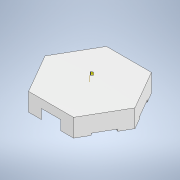
# Autodesk Inventor part: Hexagone
Saved by Autodesk Inventor 2020 (Build 240168000, 168)
## iProperties
Created: 2020-04-08
Part Number: Hexagone
Material: PVC-Piping
Document SubType Name: Modeling
Designer: Samuele
Density: 1.4 g/cm^3
Appearance: Smooth - White
Author: Samuele
## iProperties of the stored document _3DPrint.ipt
Created: 2020-04-24
Part Number: _3DPrint
Material: Generic
Document SubType Name: Modeling
Designer: Samuele
Density: 1 g/cm^3
Appearance: Default
Author: Samuele
Autodesk Inventor part; units mm, degrees
ref_plane "YZ Plane" through (0, 0, 0) normal (1, 0, 0) x (0, 1, 0)
ref_plane "XZ Plane" through (0, 0, 0) normal (0, 1, 0) x (-1, 0, 0)
ref_plane "XY Plane" through (0, 0, 0) normal (0, 0, 1) x (1, 0, 0)
sketch "Sketch6" plane through (0, 0, 0) normal (0, 1, 0) x (-1, 0, 0)
  circle A0 centre (32.5, -48.5) radius 70
  line L0 (102.5, -48.5) -> (67.5, -109.1218)
  line L1 (67.5, -109.1218) -> (-2.5, -109.1218)
  line L2 (-2.5, -109.1218) -> (-37.5, -48.5)
  line L3 (-37.5, -48.5) -> (-2.5, 12.1218)
  line L4 (-2.5, 12.1218) -> (67.5, 12.1218)
  line L5 (67.5, 12.1218) -> (102.5, -48.5)
  line L6 (32.5, 12.1218) -> (47.5, 12.1218)
  line L7 (47.5, 12.1218) -> (47.5, 5.6218)
  line L8 (47.5, 5.6218) -> (17.5, 5.6218)
  line L9 (17.5, 5.6218) -> (17.5, 12.1218)
  line L10 (47.5, 5.6218) -> (56.6924, 5.6218) construction
  line L11 (17.5, 8.8718) -> (20, 8.8718)
  line L12 (47.5, 8.8718) -> (45, 8.8718)
  line L13 (45, 8.8718) -> (45, 10.1218)
  line L14 (45, 10.1218) -> (20, 10.1218)
  line L15 (20, 10.1218) -> (20, 7.6218)
  line L16 (20, 7.6218) -> (45, 7.6218)
  line L17 (45, 7.6218) -> (45, 10.1218)
  line L18 (47.5, 5.6218) -> (56.6924, 5.6218)
  line L19 (17.5, 5.6218) -> (11, 5.6218)
  line L20 (17.5, 12.1218) -> (11, 5.6218)
  line L21 (17.5, 12.1218) -> (26.6924, 12.1218) construction
  line L22 (47.5, 12.1218) -> (54, 5.6218)
  line L23 (85, -18.1891) -> (77.5, -5.1987)
  line L24 (77.5, -5.1987) -> (71.8708, -8.4487)
  line L25 (71.8708, -8.4487) -> (86.8708, -34.4295)
  line L26 (86.8708, -34.4295) -> (92.5, -31.1795)
  line L27 (71.8708, -8.4487) -> (67.2746, -0.4879) construction
  line L28 (89.6854, -32.8045) -> (88.4354, -30.6394)
  line L29 (74.6854, -6.8237) -> (75.9354, -8.9888)
  line L30 (75.9354, -8.9888) -> (77.0179, -8.3638)
  line L31 (77.0179, -8.3638) -> (89.5179, -30.0144)
  line L32 (89.5179, -30.0144) -> (87.3529, -31.2644)
  line L33 (87.3529, -31.2644) -> (74.8529, -9.6138)
  line L34 (74.8529, -9.6138) -> (77.0179, -8.3638)
  line L35 (71.8708, -8.4487) -> (67.2746, -0.4879)
  line L36 (86.8708, -34.4295) -> (90.1208, -40.0587)
  line L37 (92.5, -31.1795) -> (90.1208, -40.0587)
  line L38 (92.5, -31.1795) -> (87.9038, -23.2187) construction
  line L39 (77.5, -5.1987) -> (68.6208, -2.8196)
  line L40 (71.8708, -88.5513) -> (67.2746, -96.5121) construction
  line L41 (74.6854, -90.1763) -> (75.9354, -88.0112)
  line L42 (74.8529, -87.3862) -> (77.0179, -88.6362)
  line L43 (77.5, -91.8013) -> (71.8708, -88.5513)
  line L44 (77.5, -91.8013) -> (68.6208, -94.1804)
  line L45 (71.8708, -88.5513) -> (67.2746, -96.5121)
  line L46 (77.0179, -88.6362) -> (89.5179, -66.9856)
  line L47 (87.3529, -65.7356) -> (74.8529, -87.3862)
  line L48 (71.8708, -88.5513) -> (86.8708, -62.5705)
  line L49 (89.5179, -66.9856) -> (87.3529, -65.7356)
  line L50 (89.6854, -64.1955) -> (88.4354, -66.3606)
  line L51 (86.8708, -62.5705) -> (92.5, -65.8205)
  line L52 (86.8708, -62.5705) -> (90.1208, -56.9413)
  line L53 (92.5, -65.8205) -> (90.1208, -56.9413)
  line L54 (94.9944, -48.5) -> (63.7472, -102.6218)
  line L55 (63.7472, -102.6218) -> (1.2528, -102.6218)
  line L56 (1.2528, -102.6218) -> (-29.9944, -48.5)
  line L57 (-29.9944, -48.5) -> (1.2528, 5.6218)
  line L58 (1.2528, 5.6218) -> (63.7472, 5.6218)
  line L59 (63.7472, 5.6218) -> (94.9944, -48.5)
  line L60 (74.8529, -87.3862) -> (73.1208, -86.3862)
  line L61 (87.3529, -65.7356) -> (85.6208, -64.7356)
  line L62 (87.3529, -31.2644) -> (85.6208, -32.2644)
  line L63 (74.8529, -9.6138) -> (73.1208, -10.6138)
  line L64 (45, 7.6218) -> (45, 5.6218)
  line L65 (20, 7.6218) -> (20, 5.6218)
  line L66 (-29.9944, -48.5) -> (-22.9944, -48.5)
  line L67 (-29.9944, -48.5) -> (-28.2944, -48.5)
  line L68 (-28.2944, -48.5) -> (-22.9944, -48.5)
  circle A1 centre (-26.9944, -48.5) radius 1.5
  line L69 (-29.9944, -48.5) -> (-23.9944, -48.5)
  line L70 (-23.9944, -48.5) -> (-26.9944, -53.6962)
  line L71 (-23.9944, -48.5) -> (-26.9944, -43.3038)
  point P0 (-27.5473, -52.7386)
  point P1 (-28.2775, -45.5261)
  point P2 (88.4354, -30.6394)
  point P3 (75.9354, -8.9888)
  point P4 (76.4767, -8.6763)
  point P5 (89.6854, -32.8045)
  point P6 (86.4869, -65.2356)
  point P7 (88.4354, -66.3606)
  dimension "d127" = 140
  dimension "d87" = 15
  dimension "d88" = 6.5
  dimension "d91" = 2.5
  dimension "d92" = 2.5
  dimension "d95" = 1.25
  dimension "d96" = 25
  dimension "d97" = 2.5
  dimension "d98" = 25
  dimension "d99" = 135
  dimension "d100" = 0
  dimension "d114" = 1.7
  dimension "d117" = 3
  dimension "d121" = 3
  dimension "d123" = 6
  dimension "d128" = 5.1962
  dimension "d129" = 5.1962
  dimension "d130" = 3
  constraints: 144 end point, 17 point on line, 9 midpoint, 8 perpendicular, 6 horizontal, 3 vertical, 2 collinear, 2 horizontal alignment, 2 parallel, 1 centre point, 1 equal length, 49 other
  measures "d87" distance of L6.start L6.end
  measures "d88" distance of L6.end L7.end
  measures "d91" distance of L11.start L11.end
  measures "d92" distance of L12.start L12.end
  measures "d95" distance of L12.end L13.end
  measures "d96" distance of L13.end L14.end
  measures "d97" distance of L14.end L15.end
  measures "d98" distance of L15.end L16.end
  measures "d99" angle of L20 L21
  measures "d100" distance of L9.end L20.start
  measures "d114" distance of L56.end L67.end
  measures "d117" diameter of A1
  measures "d121" distance of L56.end A1.centre
  measures "d123" distance of L56.end L69.end
  measures "d128" vertical distance of L69.end L70.end
  measures "d129" vertical distance of L69.end L71.end
  measures "d130" distance of L69.end A1.centre
extrude "Fronte" add sketch "Sketch6" along normal blind 3 contours L0 L53 L54 L59 L37 L5 | L5 L39 L35 L59 L58 L18 L22 L4 | L1 L2 L3 L4 L20 L58 L57 L56 L55 L54 L45 L44 L0 | L0 L43 L41 L42 L46 L49 L50 L51 | L51 L52 L53 | L26 L28 L32 L31 L30 L29 L24 L5 | L37 L36 L26 | L7 L12 L13 L14 L15 L11 L9 L4 | L22 L18 L7 | L24 L35 L39 | L44 L45 L43 | L50 L49 L61 L48 L51 | L52 L48 L45 L54 L55 L56 L70 L71 L57 L58 L19 L8 L18 L59 L35 L25 L36 | L26 L25 L62 L32 L28 | L9 L19 L20 | L7 L8 L64 L17 L12 | L29 L34 L63 L25 L24 | L43 L48 L60 L42 L41 | L49 L46 L42 L47 | L32 L33 L34 L30 L31 | L11 L15 L65 L8 L9 | L17 L16 L15 L14 L13 | L47 L60 L48 L61 | L25 L63 L33 L62 | L8 L65 L16 L64 | L71 L66 A1 L57 | L66 A1 L70 L56 | A1 L66 | L66 A1
extrude "Esterno" add sketch "Sketch6" against normal blind 25 contours L0 L53 L54 L59 L37 L5 | L5 L39 L35 L59 L58 L18 L22 L4 | L1 L2 L3 L4 L20 L58 L57 L56 L55 L54 L45 L44 L0
extrude "Strip" add sketch "Sketch6" against normal blind 10 contours L0 L43 L41 L42 L46 L49 L50 L51 | L51 L52 L53 | L26 L28 L32 L31 L30 L29 L24 L5 | L37 L36 L26 | L7 L12 L13 L14 L15 L11 L9 L4 | L22 L18 L7 | L24 L35 L39 | L44 L45 L43 | L50 L49 L61 L48 L51 | L26 L25 L62 L32 L28 | L9 L19 L20 | L7 L8 L64 L17 L12 | L29 L34 L63 L25 L24 | L43 L48 L60 L42 L41 | L11 L15 L65 L8 L9 | L47 L60 L48 L61 | L25 L63 L33 L62 | L8 L65 L16 L64
sketch "Sketch7" plane through (0, -25, 0) normal (0, -1, 0) x (1, 0, 0)
  line L0 (-17.5, 12.1218) -> (-17.5, -109.1218)
  line L1 (-67.5, -109.1218) -> (2.5, -109.1218) projected
  line L2 (-47.5, 12.1218) -> (-67.5, 12.1218) projected
  line L3 (-47.5, 12.1218) -> (-47.5, -109.1218)
  line L4 (-77.5, -91.8013) -> (-67.5, -109.1218) projected
  line L5 (-77.5, -91.8013) -> (27.5, -31.1795)
  line L6 (2.5, 12.1218) -> (37.5, -48.5) projected
  line L7 (-92.5, -65.8205) -> (-90.1208, -56.9413) projected
  line L8 (-92.5, -65.8205) -> (12.5, -5.1987)
  line L9 (-77.5, -5.1987) -> (27.5, -65.8205)
  line L10 (37.5, -48.5) -> (2.5, -109.1218) projected
  line L11 (-92.5, -31.1795) -> (11.423, -93.6666)
  line L12 (27.5, -31.1795) -> (12.5, -5.1987)
  line L13 (27.5, -65.8205) -> (11.423, -93.6666)
  line L14 (-1.2528, -102.6218) -> (29.9944, -48.5) projected
  line L15 (5.8516, -90.3166) -> (21.8708, -62.5705)
  line L16 (-47.5, -109.1218) -> (-17.5, -109.1218)
  line L17 (-17.5, -109.1218) -> (-17.5, -102.6218)
  line L18 (-17.5, -102.6218) -> (-47.5, -102.6218)
  line L19 (-47.5, -102.6218) -> (-47.5, -109.1218)
  line L20 (5.5339, -9.2206) -> (17.5, -36.953)
  point P0 (0, 0)
  point P1 (6.9325, -8.4131)
  point P2 (21.9325, -34.3939)
  constraints: 28 end point, 13 point on line, 3 parallel, 2 vertical, 1 horizontal, 1 perpendicular
extrude "Passacavi" cut sketch "Sketch7" against normal blind 3 contours L0 L1 L3 L18 | L14 L9 L10 L11 | L20 L8 L6 L5
extrude "ScavoStrip" cut sketch "Sketch6" against normal blind 5 contours L47 L60 L48 L61 | L25 L63 L33 L62 | L8 L65 L16 L64
extrude "SupportoViti" add sketch "Sketch6" against normal blind 23 contours L71 L66 A1 L57 | L66 A1 L70 L56
pattern_circular "RipetizioneFori" count 6 over 360 about axis through (-32.5, 0, -48.5) along (0, 1, 0) of "SupportoViti"
sketch "Sketch10" plane through (0, 0, 0) normal (0, -1, 0) x (1, 0, 0)
  line L0 (-11, 5.6218) -> (-1.2528, 5.6218) projected
  line L1 (-63.7472, -102.6218) -> (-68.6208, -94.1804) projected
  line L2 (-1.2528, 5.6218) -> (-63.7472, -102.6218)
  circle A0 centre (-32.5, -48.5) radius 35
  circle A1 centre (-32.5, -48.5) radius 22.5
  circle A2 centre (-32.5, -48.5) radius 10
  line L3 (-32.5, -48.5) -> (-32.5, -83.5)
  line L4 (-32.5, -48.5) -> (-37.0684, -83.2006)
  line L5 (-32.5, -48.5) -> (2.5, -48.5) construction
  line L6 (-32.5, -48.5) -> (-27.9316, -83.2006)
  line L7 (-32.5, -83.5) -> (-32.5, -13.5)
  line L8 (2.5, -48.5) -> (-67.5, -48.5)
  line L9 (-32.5, -48.5) -> (-37.0684, -13.7994)
  line L10 (-32.5, -48.5) -> (-27.9316, -13.7994)
  line L11 (-32.5, -48.5) -> (-7.7513, -73.2487)
  line L12 (-32.5, -48.5) -> (2.5, -48.5) construction
  line L13 (-32.5, -48.5) -> (2.2006, -43.9316)
  line L14 (-32.5, -48.5) -> (2.2006, -53.0684)
  line L15 (-32.5, -48.5) -> (-67.2006, -43.9316)
  line L16 (-32.5, -48.5) -> (-67.2006, -53.0684)
  point P0 (0, 0)
  point P1 (-29.5632, -70.8075)
  point P2 (-10.1925, -51.4368)
  point P3 (-54.8075, -51.4368)
  point P4 (-35.4368, -70.8075)
  point P5 (-54.8075, -45.5632)
  point P6 (-35.4368, -26.1925)
  point P7 (-10.1925, -45.5632)
  point P8 (-29.5632, -26.1925)
  dimension "d140" = 70
  dimension "d141" = 45
  dimension "d142" = 20
  dimension "d145" = 7.5
  dimension "d146" = 45
  constraints: 30 end point, 6 symmetric about line, 5 point on circle, 3 centre point, 3 equal length, 2 coincident, 2 horizontal, 2 vertical, 1 midpoint, 1 perpendicular, 1 other
  measures "d140" diameter of A0
  measures "d141" diameter of A1
  measures "d142" diameter of A2
  measures "d145" angle of L4 L3
  measures "d146" angle of L11 L12
extrude "LightMembrane" cut sketch "Sketch10" against normal blind 2.5 contours A0 L13 A1 L2 | L2 A1 L10 A0 | A2 L13 L2 | L2 L10 A2 | L4 A2 L2 | L6 A2 L3 | L3 A2 L4 | L11 A2 L6 | L9 A2 L7 | L13 A2 L8 | L16 A2 L8 | L15 A2 L9 | L7 A2 L10 | L14 A2 L11 | L8 A2 L14 | L8 A2 L15 | L2 A2 L16 | A0 L11 A1 L14 | L9 A1 L15 A0 | A0 L6 A1 L11 | A1 L4 A0 L2 | L2 A0 L16 A1
body "Solid3"
